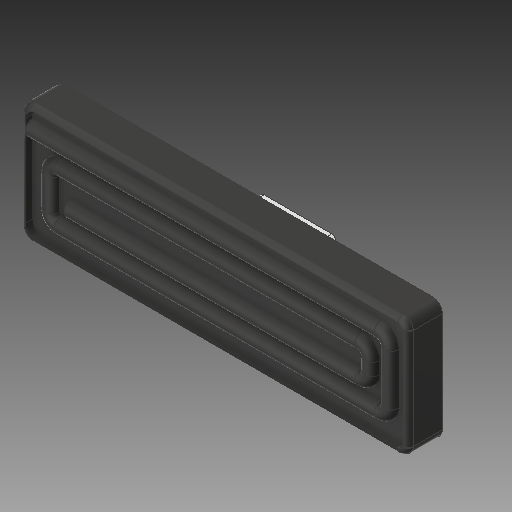
# Autodesk Inventor part: resistencia_600w
Saved by Autodesk Inventor 2018 (Build 220112000, 112)
## iProperties
Created: 2018-05-03
Part Number: resistencia_600w
Material: Genérico
Document SubType Name: Modeling
Designer: Georgines
Density: 1 g/cm^3
Appearance: Padrão
Mass: 260.3 g
Surface Area: 413.512 cm^2
Volume: 260.3 cm^3
Author: Georgines
Autodesk Inventor part; units mm, degrees
ref_plane "YZ Plane" through (0, 0, 0) normal (1, 0, 0) x (0, 1, 0)
ref_plane "XZ Plane" through (0, 0, 0) normal (0, 1, 0) x (-1, 0, 0)
ref_plane "XY Plane" through (0, 0, 0) normal (0, 0, 1) x (1, 0, 0)
sketch "Esboço1" plane through (0, 0, 0) normal (0, 0, 1) x (1, 0, 0)
  line L0 (-17.5, -7.85) -> (17.5, -7.85)
  line L1 (19.5, -5.85) -> (19.5, 5.85)
  line L2 (17.5, 7.85) -> (-17.5, 7.85)
  line L3 (-19.5, 5.85) -> (-19.5, -5.85)
  line L4 (-19.5, -7.85) -> (19.5, 7.85) construction
  line L5 (19.5, -7.85) -> (-19.5, 7.85) construction
  arc A0 (-17.5, 7.85) -> (-19.5, 5.85) centre (-17.5, 5.85) ccw
  arc A1 (-19.5, -5.85) -> (-17.5, -7.85) centre (-17.5, -5.85) ccw
  arc A2 (19.5, 5.85) -> (17.5, 7.85) centre (17.5, 5.85) ccw
  arc A3 (17.5, -7.85) -> (19.5, -5.85) centre (17.5, -5.85) ccw
  point P0 (0, 0)
  dimension "d0" = 39
  dimension "d1" = 15.7
  dimension "d2" = 2
  constraints: 12 end point, 8 point on circle, 8 point on line, 8 tangent, 4 centre point, 3 equal radius, 2 midpoint, 2 parallel, 1 horizontal, 1 perpendicular
  measures "d0" distance of L5.end L4.end
  measures "d1" distance of L4.end L5.start
  measures "d2" radius of A0
extrude "Extrusão1" add sketch "Esboço1" along normal blind 13.35
sketch "Esboço2" plane through (0, 0, 13.35) normal (0, 0, 1) x (1, 0, 0)
  line L0 (-23, 13.15) -> (23, 13.15)
  line L1 (25, 11.15) -> (25, -11.15)
  line L2 (23, -13.15) -> (-23, -13.15)
  line L3 (-25, -11.15) -> (-25, 11.15)
  line L4 (-25, 13.15) -> (25, -13.15) construction
  line L5 (25, 13.15) -> (-25, -13.15) construction
  arc A0 (-23, 13.15) -> (-25, 11.15) centre (-23, 11.15) ccw
  arc A1 (-25, -11.15) -> (-23, -13.15) centre (-23, -11.15) ccw
  arc A2 (23, -13.15) -> (25, -11.15) centre (23, -11.15) ccw
  arc A3 (25, 11.15) -> (23, 13.15) centre (23, 11.15) ccw
  point P0 (0, 0)
  dimension "d5" = 50
  dimension "d6" = 26.3
  dimension "d7" = 2
  constraints: 12 end point, 8 point on circle, 8 point on line, 8 tangent, 4 centre point, 3 equal radius, 2 midpoint, 2 parallel, 1 horizontal, 1 perpendicular
  measures "d5" distance of L4.end L5.end
  measures "d6" distance of L5.start L4.end
  measures "d7" radius of A0
extrude "Extrusão2" add sketch "Esboço2" along normal blind 4.42
sketch "Esboço3" plane through (0, 0, 17.77) normal (0, 0, 1) x (1, 0, 0)
  line L0 (-40.3, 13.15) -> (40.3, 13.15)
  line L1 (42.3, 11.15) -> (42.3, -11.15)
  line L2 (40.3, -13.15) -> (-40.3, -13.15)
  line L3 (-42.3, -11.15) -> (-42.3, 11.15)
  line L4 (-42.3, 13.15) -> (42.3, -13.15) construction
  line L5 (42.3, 13.15) -> (-42.3, -13.15) construction
  arc A0 (42.3, 11.15) -> (40.3, 13.15) centre (40.3, 11.15) ccw
  arc A1 (40.3, -13.15) -> (42.3, -11.15) centre (40.3, -11.15) ccw
  arc A2 (-42.3, -11.15) -> (-40.3, -13.15) centre (-40.3, -11.15) ccw
  arc A3 (-40.3, 13.15) -> (-42.3, 11.15) centre (-40.3, 11.15) ccw
  point P0 (0, 0)
  dimension "d10" = 84.6
  dimension "d18" = 2
  constraints: 12 end point, 8 point on circle, 8 point on line, 8 tangent, 4 centre point, 3 equal radius, 2 midpoint, 2 parallel, 1 horizontal, 1 perpendicular
  measures "d10" distance of L4.end L5.end
  measures "d18" radius of A0
ref_plane "Plano de trabalho2" through (0, 0, 25.27) normal (0, 0, 1) x (1, 0, 0)
sketch "Esboço5" plane through (0, 0, 25.27) normal (0, 0, 1) x (1, 0, 0)
  line L0 (95, -31) -> (-95, -31)
  line L1 (-100, -26) -> (-100, 26)
  line L2 (-95, 31) -> (95, 31)
  line L3 (100, 26) -> (100, -26)
  line L4 (100, -31) -> (-100, 31) construction
  line L5 (-100, -31) -> (100, 31) construction
  arc A0 (-100, -26) -> (-95, -31) centre (-95, -26) ccw
  arc A1 (-95, 31) -> (-100, 26) centre (-95, 26) ccw
  arc A2 (95, -31) -> (100, -26) centre (95, -26) ccw
  arc A3 (100, 26) -> (95, 31) centre (95, 26) ccw
  point P0 (0, 0)
  dimension "d21" = 200
  dimension "d22" = 62
  dimension "d25" = 5
  constraints: 12 end point, 8 point on circle, 8 point on line, 8 tangent, 4 centre point, 3 equal radius, 2 midpoint, 2 parallel, 1 horizontal, 1 perpendicular
  measures "d21" distance of L4.end L5.end
  measures "d22" distance of L5.start L4.end
  measures "d25" radius of A0
extrude "Extrusão5" add sketch "Esboço5" along normal blind 14.05
loft "Transição1" add profiles "Esboço3" section 2 edges at (-100, 0, 25.27) (-98.5355, 29.5355, 25.27) (0, 31, 25.27) (98.5355, 29.5355, 25.27) (100, 0, 25.27) (98.5355, -29.5355, 25.27) (0, -31, 25.27) (-98.5355, -29.5355, 25.27)
sketch "Esboço6" plane through (0, 0, 39.32) normal (0, 0, 1) x (1, 0, 0)
  line L0 (-95, -31) -> (95, -31)
  line L1 (100, -26) -> (100, 26)
  line L2 (95, 31) -> (-95, 31)
  line L3 (-100, 26) -> (-100, -26)
  line L4 (-100, -31) -> (100, 31) construction
  line L5 (100, -31) -> (-100, 31) construction
  line L6 (-92.75, 28.5) -> (92.75, 28.5)
  line L7 (97.75, 23.5) -> (97.75, -23.5)
  line L8 (92.75, -28.5) -> (-92.75, -28.5)
  line L9 (-97.75, -23.5) -> (-97.75, 23.5)
  line L10 (-97.75, 28.5) -> (97.75, -28.5) construction
  line L11 (97.75, 28.5) -> (-97.75, -28.5) construction
  arc A0 (-100, -26) -> (-95, -31) centre (-95, -26) ccw
  arc A1 (-95, 31) -> (-100, 26) centre (-95, 26) ccw
  arc A2 (100, 26) -> (95, 31) centre (95, 26) ccw
  arc A3 (95, -31) -> (100, -26) centre (95, -26) ccw
  arc A4 (92.75, -28.5) -> (97.75, -23.5) centre (92.75, -23.5) ccw
  arc A5 (97.75, 23.5) -> (92.75, 28.5) centre (92.75, 23.5) ccw
  arc A6 (-92.75, 28.5) -> (-97.75, 23.5) centre (-92.75, 23.5) ccw
  arc A7 (-97.75, -23.5) -> (-92.75, -28.5) centre (-92.75, -23.5) ccw
  line L12 (-97.75, 19.798) -> (11.75, 19.798)
  line L13 (11.75, 19.798) -> (11.75, -18.5)
  line L14 (11.75, -18.5) -> (-87.75, -18.5)
  line L15 (-87.75, -18.5) -> (-87.75, 9.798)
  line L16 (-87.75, 9.798) -> (1.75, 9.798)
  line L17 (1.75, 9.798) -> (1.75, -8.5)
  line L18 (1.75, -8.5) -> (-77.75, -8.5)
  line L19 (-77.75, -8.5) -> (-77.75, -0.202)
  line L20 (-77.75, -0.202) -> (-8.25, -0.202)
  point P0 (0, 0)
  dimension "d30" = 195.5
  dimension "d31" = 57
  dimension "d32" = 5
  dimension "d46" = 109.5
  dimension "d47" = 38.298
  dimension "d48" = 99.5
  dimension "d49" = 28.298
  dimension "d50" = 89.5
  dimension "d51" = 18.298
  dimension "d52" = 79.5
  dimension "d53" = 8.298
  dimension "d54" = 69.5
  dimension "d69" = 200
  dimension "d70" = 62
  constraints: 42 end point, 17 point on line, 16 point on circle, 16 tangent, 10 perpendicular, 8 centre point, 7 equal radius, 5 parallel, 4 midpoint, 2 horizontal
  measures "d30" distance of L10.end L11.end
  measures "d31" distance of L11.start L10.end
  measures "d32" radius of A0
  measures "d46" distance of L12.start L12.end
  measures "d47" distance of L12.end L13.end
  measures "d48" distance of L13.end L14.end
  measures "d49" distance of L14.end L15.end
  measures "d50" distance of L15.end L16.end
  measures "d51" distance of L16.end L17.end
  measures "d52" distance of L17.end L18.end
  measures "d53" distance of L18.end L19.end
  measures "d54" distance of L19.end L20.end
  measures "d69" distance between parallel lines of L1 L3
  measures "d70" distance between parallel lines of L0 L2
extrude "Extrusão6" add sketch "Esboço6" along normal blind 4
ref_plane "Plano de trabalho4" through (0, 0, 39.32) normal (0, 0, 1) x (1, 0, 0)
sketch "Esboço10" plane through (0, 0, 39.32) normal (0, 0, 1) x (1, 0, 0)
  line L0 (-97.75, 23.5) -> (-97.75, -23.5) projected
  line L1 (-97.6618, 17.8549) -> (6.8382, 17.8549)
  line L2 (6.8382, 17.8549) -> (82.7502, 17.8549)
  line L3 (87.7502, 12.8549) -> (87.7502, -13.5001)
  line L4 (82.7502, -18.5001) -> (-82.7498, -18.5001)
  line L5 (-87.7498, -13.5001) -> (-87.7498, 2.8549)
  line L6 (-82.7498, 7.8549) -> (72.7502, 7.8549)
  line L7 (77.7502, 2.8549) -> (77.7502, -3.5001)
  line L8 (72.7502, -8.5001) -> (-77.7498, -8.5001)
  arc A0 (87.7502, 12.8549) -> (82.7502, 17.8549) centre (82.7502, 12.8549) ccw
  arc A1 (82.7502, -18.5001) -> (87.7502, -13.5001) centre (82.7502, -13.5001) ccw
  arc A2 (-87.7498, -13.5001) -> (-82.7498, -18.5001) centre (-82.7498, -13.5001) ccw
  arc A3 (-82.7498, 7.8549) -> (-87.7498, 2.8549) centre (-82.7498, 2.8549) ccw
  arc A4 (77.7502, 2.8549) -> (72.7502, 7.8549) centre (72.7502, 2.8549) ccw
  arc A5 (72.7502, -8.5001) -> (77.7502, -3.5001) centre (72.7502, -3.5001) ccw
  point P0 (0, 0)
  point P1 (87.7502, 17.8549)
  point P2 (87.7502, -18.5001)
  point P3 (-87.7498, -18.5001)
  point P4 (-87.7498, 7.8549)
  point P5 (77.7502, 7.8549)
  point P6 (77.7502, -8.5001)
  dimension "d71" = 80.912
  dimension "d72" = 36.355
  dimension "d73" = 175.5
  dimension "d74" = 26.355
  dimension "d75" = 165.5
  dimension "d76" = 16.355
  dimension "d77" = 155.5
  dimension "d78" = 5
  constraints: 16 end point, 12 point on circle, 12 point on line, 12 tangent, 7 perpendicular, 6 centre point, 5 equal radius, 2 horizontal
  measures "d71" distance of L1.end point (87.75, 17.855)
  measures "d72" distance of point (87.75, 17.855) point (87.75, -18.5)
  measures "d73" distance of point (87.75, -18.5) point (-87.75, -18.5)
  measures "d74" distance of point (-87.75, -18.5) point (-87.75, 7.855)
  measures "d75" distance of point (-87.75, 7.855) point (77.75, 7.855)
  measures "d76" distance of point (77.75, 7.855) point (77.75, -8.5)
  measures "d77" distance of point (77.75, -8.5) L8.end
  measures "d78" radius of A0
fillet "Arredondamento2" radius 3 1 edges at (0, -31, 43.32)
ref_plane "Plano de trabalho6" through (-77.7498, -8.5001, 39.32) normal (-1, 0, 0) x (0, -1, 0)
sketch "Esboço12" plane through (-77.7498, -8.5001, 39.32) normal (-1, 0, 0) x (0, -1, 0)
  arc A0 (3.9998, -0.0383) -> (-3.9998, -0.0383) centre (0, 0) ccw
  line L0 (-3.9998, -0.0383) -> (3.9998, -0.0383)
  line L1 (14.9999, 3.9047) -> (-32.0001, 3.9047) projected
  point P0 (-8.5001, -39.32)
  dimension "d79" = 8
  constraints: 2 end point, 2 point on circle, 1 centre point, 1 horizontal, 1 other
  measures "d79" diameter of A0
sweep "Varredura2" add profiles "Esboço12" path "Esboço10" path curves L8 A5 L7 A4 L6 A3 L5 A2 L4 A1 L3 A0 L2 L1
